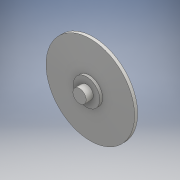
# Autodesk Inventor part: enlacecuello
Saved by Autodesk Inventor 2016 (Build 200138000, 138)
## iProperties
Created: 2016-02-20
Part Number: enlacecuello
Material: Genérico
Document SubType Name: Modeling
Designer: Usuario1
Density: 1 g/cm^3
Appearance: Valor por defecto
Author: Usuario1
Autodesk Inventor part; units mm, degrees
ref_plane "YZ Plane" through (0, 0, 0) normal (1, 0, 0) x (0, 1, 0)
ref_plane "XZ Plane" through (0, 0, 0) normal (0, 1, 0) x (-1, 0, 0)
ref_plane "XY Plane" through (0, 0, 0) normal (0, 0, 1) x (1, 0, 0)
sketch "Boceto1" plane through (0, 0, 0) normal (0, 0, 1) x (1, 0, 0)
  line L0 (0, 1.5671) -> (-5, 1.5671)
  line L1 (-5, 1.5671) -> (-5, 1.2168)
  line L2 (-1.5, 1.1) -> (-5, 1.2168)
  line L3 (-1.5, 1.1) -> (-1.5, 0.8)
  line L4 (-1.5, 0.8) -> (-0.75, 0.8)
  line L5 (-0.75, 0.8) -> (-0.75, 0)
  line L6 (-0.75, 0) -> (0, 0)
  line L7 (0, 0) -> (0, 1.5671)
  constraints: 16 end point
revolve "Revolución1" add sketch "Boceto1" angle 360 about axis through (0, 0, 0) along (0, 1, 0)
sketch "Boceto2" plane through (0, 1.5671, 0) normal (0, 1, 0) x (1, 0, 0)
  line L0 (0, 0) -> (-0.75, 0)
  circle A0 centre (0, 0) radius 0.75 projected
  line L1 (-0.75, 0) -> (-0.75, 0.75)
  line L2 (-0.75, 0.75) -> (0.75, 0.75)
  line L3 (0.75, 0.75) -> (0.75, -0.75)
  line L4 (0.75, -0.75) -> (-0.75, -0.75)
  line L5 (-0.75, -0.75) -> (-0.75, 0)
  dimension "d1" = 0.75
  dimension "d2" = 0.75
  dimension "d3" = 1.5
  dimension "d4" = 1.5
  dimension "d5" = 1.5
  constraints: 12 end point, 2 horizontal, 2 perpendicular, 1 tangent
  measures "d1" distance of L0.start L0.end
  measures "d2" distance of L0.end L1.end
  measures "d3" distance of L1.end L2.end
  measures "d4" distance of L2.end L3.end
  measures "d5" distance of L3.end L4.end
extrude "Extrusión1" add sketch "Boceto2" along normal blind 0.8
